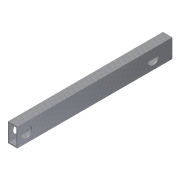
# Autodesk Inventor part: Frame Side
Saved by Autodesk Inventor 2011 (Build 150239000, 239)
## iProperties
Created: 2014-09-13
Part Number: Frame Side
Document SubType Name: Modeling
Designer: Family Room
Density: 1 g/cm^3
Author: Family Room
Autodesk Inventor part; units mm, degrees
ref_plane "YZ Plane" through (0, 0, 0) normal (1, 0, 0) x (0, 1, 0)
ref_plane "XZ Plane" through (0, 0, 0) normal (0, 1, 0) x (-1, 0, 0)
ref_plane "XY Plane" through (0, 0, 0) normal (0, 0, 1) x (1, 0, 0)
sketch "Sketch1" plane through (0, 0, 0) normal (0, 0, 1) x (1, 0, 0)
  line L0 (0, 0) -> (25.4, 0)
  line L1 (25.4, 0) -> (25.4, 50.8)
  line L2 (25.4, 50.8) -> (0, 50.8)
  line L3 (0, 50.8) -> (0, 0)
  line L4 (3.175, 47.625) -> (22.225, 47.625)
  line L5 (22.225, 47.625) -> (22.225, 3.175)
  line L6 (22.225, 3.175) -> (3.175, 3.175)
  line L7 (3.175, 3.175) -> (3.175, 47.625)
  dimension "d0" = 25.4
  dimension "d1" = 50.8
  dimension "d2" = 3.175
  constraints: 16 end point, 4 parallel, 2 perpendicular, 1 horizontal, 3 other
  measures "d0" distance of L2.end L1.end
  measures "d1" distance of L1.end L0.end
  measures "d2" distance between parallel lines of L2 L4
extrude "Extrusion1" add sketch "Sketch1" along normal blind 419.1
sketch "Sketch2" plane through (25.4, 0, 0) normal (1, 0, 0) x (0, 0, -1)
  line L0 (-419.1, 50.8) -> (-419.1, 0) projected
  line L1 (0, 0) -> (0, 50.8) projected
  line L2 (0, 50.8) -> (-419.1, 50.8) projected
  point P0 (-393.7, 25.4)
  point P1 (-50.8, 25.4)
  dimension "d5" = 25.4
  dimension "d6" = 25.4
  dimension "d7" = 50.8
  measures "d5" distance from line of L0 point (-393.7, 25.4)
  measures "d6" distance from line of L2 point (-393.7, 25.4)
  measures "d7" distance from line of L1 point (-50.8, 25.4)
hole "Hole1" at (25.4, 25.4, 393.7) at (25.4, 25.4, 50.8) direction (-1, 0, 0) diameter 28.575 depth 25.4 tip angle 118
ref_plane "Work Plane1" through (0, 0, 209.55) normal (0, 0, 1) x (1, 0, 0)
ref_plane "Work Plane2" through (12.7, 0, 0) normal (1, 0, 0) x (0, 0, -1)
ref_plane "Work Plane3" through (0, 0, 304.8) normal (0, 0, 1) x (1, 0, 0)
body "Solid1"
